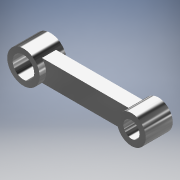
# Autodesk Inventor part: rod
Saved by Autodesk Inventor 2018.1 (Build 221171000, 171)
## iProperties
Created: 2013-08-27
Part Number: rod
Material: Generic
Document SubType Name: Modeling
Designer: Konstantin
Density: 1 g/cm^3
Appearance: Default
Mass: 0.308147 g
Surface Area: 5.27976 cm^2
Volume: 0.308147 cm^3
Author: Konstantin
Autodesk Inventor part; units mm, degrees
ref_plane "YZ Plane" through (0, 0, 0) normal (1, 0, 0) x (0, 1, 0)
ref_plane "XZ Plane" through (0, 0, 0) normal (0, 1, 0) x (-1, 0, 0)
ref_plane "XY Plane" through (0, 0, 0) normal (0, 0, 1) x (1, 0, 0)
sketch "Sketch1" plane through (0, 0, 0) normal (0, 0, 1) x (1, 0, 0)
  circle A0 centre (0, 0) radius 2
  circle A1 centre (20, 0) radius 1.5
  arc A2 (18.2615, -2) -> (18.2615, 2) centre (20, 0) ccw
  arc A3 (2.2361, 2) -> (2.2361, -2) centre (0, 0) ccw
  line L0 (2.2361, -2) -> (18.2615, -2)
  line L1 (2.2361, 2) -> (18.2615, 2)
  constraints: 4 centre point, 4 end point, 4 point on circle, 3 coincident, 2 horizontal, 1 parallel, 4 other
extrude "Extrusion1" add sketch "Sketch1" along normal mid plane 2.6
sketch "Sketch2" plane through (0, 0, 1.3) normal (0, 0, 1) x (1, 0, 0)
  circle A0 centre (0, 0) radius 3
  circle A1 centre (0, 0) radius 2
  circle A2 centre (20, 0) radius 2.65
  circle A3 centre (20, 0) radius 1.5
  constraints: 4 centre point, 4 other
extrude "Extrusion2" add sketch "Sketch2" along normal blind 1.2
mirror "Mirror1" about plane through (0, 0, 0) normal (0, 0, 1) of "Extrusion2"
ref_plane "Work Plane1" through (0, 0, 0) normal (0, 0, 1) x (1, 0, 0)
body "Solid1"
